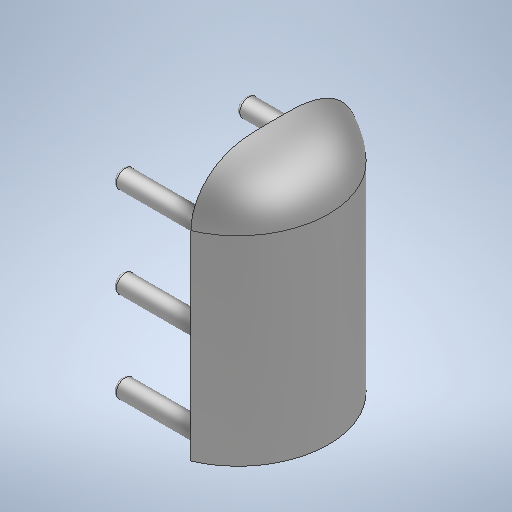
# Autodesk Inventor part: Pot Side
Saved by Autodesk Inventor 2025.2 (Build 292293000, 293)
## iProperties
Created: 2025-02-16
Part Number: Pot Side
Material: Generic
Document SubType Name: Modeling
Designer: eason
Density: 1 g/cm^3
Appearance: Anodized - Light Gray
Author: eason
Autodesk Inventor part; units mm, degrees
ref_plane "XZ Plane" through (0, 0, 0) normal (0, 1, 0) x (-1, 0, 0)
sketch "Sketch1" plane through (0, 0, 0) normal (0, 0, 1) x (1, 0, 0)
  line L0 (0, 0) -> (0, 70)
  line L1 (0, 0) -> (25, 0)
  line L2 (25, 0) -> (25, 55)
  line L3 (0, -14.6213) -> (0, 87.7279) projected
  line L4 (0, 70) -> (10, 70)
  arc A0 (25, 55) -> (10, 70) centre (10, 55) ccw
  dimension "d0" = 70
  dimension "d1" = 25
  dimension "d2" = 10
  constraints: 8 end point, 2 point on circle, 2 tangent, 2 vertical, 1 centre point, 1 horizontal, 1 perpendicular
  measures "d0" distance of L0.start L0.end
  measures "d1" distance of L0.start L1.end
  measures "d2" distance of L0.end L4.end
revolve "Revolution1" add sketch "Sketch1" angle 360 about axis through (0, -10, 0) along (0, 1, 0)
sketch "Sketch2" plane through (0, 0, 0) normal (0, -1, 0) x (1, 0, 0)
  circle A0 centre (0, 0) radius 10
  dimension "d4" = 20
  constraints: 1 centre point, 1 coincident
  measures "d4" diameter of A0
extrude "Extrusion1" cut sketch "Sketch2" against normal blind 25
sketch "Sketch3" plane through (0, 70, 0) normal (0, 1, 0) x (1, 0, 0)
  circle A0 centre (0, 0) radius 10 projected
  line L0 (10, 0) -> (-10, 0) construction
  line L1 (-35, 0) -> (35, 0) construction
  constraints: 2 end point, 2 point on circle, 1 collinear
ref_plane "Work Plane1" through (10, 70, 0) normal (1, 0, 0) x (0, 1, 0)
ref_plane "Work Plane2" through (-10, 70, 0) normal (1, 0, 0) x (0, 1, 0)
ref_plane "Work Plane3" through (0, 27.5, 25) normal (0, 0, 1) x (1, 0, 0)
sketch "Sketch4" plane through (0, 27.5, 25) normal (0, 0, 1) x (1, 0, 0)
  line L0 (10, 56.5) -> (10, -41.5) projected
  line L1 (10, 42.5) -> (-10, 42.5) projected
  arc A0 (-10, 42.5) -> (-25, 27.5) centre (-10, 27.5) ccw projected
  line L2 (-25, -27.5) -> (-25, 27.5) projected
  line L3 (25, -27.5) -> (-25, -27.5) projected
  point P0 (0, -27.5)
  point P1 (10, -27.5)
extrude "Extrusion2" cut sketch "Sketch4" against normal through all
sketch "Sketch5" plane through (10, 70, 0) normal (1, 0, 0) x (0, 1, 0)
  arc A0 (-26.2642, -10) -> (-26.2642, 10) centre (-20, 0) ccw
  line L0 (-26.2642, -10) -> (-45, -10)
  line L1 (-26.2642, 10) -> (-45, 10)
  line L2 (-84.0012, 0) -> (14.0074, 0) projected
  line L3 (-70, 22.9129) -> (-70, -22.9129) projected
  line L4 (-40.2, 0) -> (-8.2, 0) construction
  line L5 (-45, -10) -> (-45, 10)
  point P0 (-70, 0)
  dimension "d10" = 23.6
  dimension "d11" = 20
  dimension "d13" = 10
  dimension "d14" = 50
  dimension "d20" = 25
  constraints: 8 end point, 3 point on circle, 2 collinear, 2 horizontal, 1 centre point, 1 parallel, 1 point on line
  measures "d10" diameter of A0
  measures "d11" distance between parallel lines of L1 L0
  measures "d13" distance between parallel lines of L2 L0
  measures "d14" distance from line of A0.centre L3
  measures "d20" distance from line of L3 L1.end
extrude "Extrusion3" cut sketch "Sketch5" along normal blind 10
sketch "Sketch7" plane through (20, 70, 0) normal (-1, 0, 0) x (0, 0, 1)
  arc A0 (10, -26.2642) -> (-10, -26.2642) centre (0, -20) ccw projected
  circle A1 centre (0, -20) radius 11.8
  line L0 (-10, -45) -> (-10, -26.2642) projected
  line L1 (10, -26.2642) -> (10, -45) projected
  arc A2 (-10, -29.51) -> (10, -29.51) centre (0, -20) ccw
  point P0 (0, -70)
  point P1 (-10, -26.2642)
  dimension "d22" = 2
  constraints: 2 centre point, 2 concentric, 2 point on circle, 2 point on line, 1 coincident
  measures "d22" radial gap between concentric circles of A2 A1
extrude "Extrusion4" add sketch "Sketch7" along normal blind 3 contours L1 A2 L0 A1
fillet "Fillet1" radius 2 4 edges at (15, 25, -10) (15, 25, 10) (10, 25, -5) (10, 25, 5)
fillet "Fillet2" radius 1 2 edges at (17, 38.2, 0) (17, 36.2, 0)
sketch "Sketch8" plane through (0, 0, 0) normal (0, -1, 0) x (1, 0, 0)
  line L0 (10, 22.9129) -> (10, -22.9129) projected
  line L1 (10, 17) -> (15, 17)
  line L2 (15, 17) -> (15, -17)
  line L3 (15, -17) -> (10, -17)
  line L4 (10, -17) -> (10, 17)
  line L5 (-17, 0) -> (32, 0) projected
  line L6 (10, 10) -> (15, 10)
  line L7 (15, 10) -> (15, -10)
  line L8 (15, -10) -> (10, -10)
  line L9 (10, -10) -> (10, 10)
  point P0 (0, 0)
  point P1 (15, 0)
  point P2 (15, 0)
  dimension "d27" = 5
  dimension "d28" = 17
  dimension "d29" = 20
  constraints: 16 end point, 4 parallel, 4 point on line, 2 horizontal, 2 midpoint, 2 perpendicular, 1 collinear
  measures "d27" distance between parallel lines of L0 L2
  measures "d28" distance between parallel lines of L5 L1
  measures "d29" distance between parallel lines of L8 L6
sketch "Sketch9" plane through (10, 0, -22.9129) normal (-1, 0, 0) x (0, 0, 1)
  line L0 (39.9129, 0) -> (39.9129, 2.5) construction
  circle A0 centre (39.9129, 2.5) radius 2.5
  line L1 (45.8258, 0) -> (0, 0) projected
  line L2 (22.9129, -14.0012) -> (22.9129, 84.0074) projected
  circle A1 centre (5.9129, 2.5) radius 2.5
  circle A2 centre (39.9129, 27.5) radius 2.5
  circle A3 centre (5.9129, 27.5) radius 2.5
  circle A4 centre (39.9129, 52.5) radius 2.5
  circle A5 centre (5.9129, 52.5) radius 2.5
  point P0 (22.9129, 0)
  point P1 (5.9129, 0)
  dimension "d31" = 5
  dimension "d47" = 34
  dimension "d50" = 25
  constraints: 6 centre point, 2 end point, 2 vertical, 1 coincident, 1 horizontal, 1 tangent, 10 other
  measures "d31" diameter of A0
  measures "d47" distance of A0.centre A1.centre
  measures "d50" distance of A0.centre A2.centre
extrude "Extrusion5" add sketch "Sketch9" along normal blind 25
fillet "Fillet3" radius 1 6 edges at (-15, 2.5, 14.5) (-15, 2.5, -19.5) (-15, 27.5, -19.5) (-15, 27.5, 14.5) (-15, 52.5, 14.5) (-15, 52.5, -19.5)
sketch "Sketch10" plane through (0, 0, 0) normal (0, -1, 0) x (1, 0, 0)
  circle A0 centre (0, 0) radius 13
  dimension "d42" = 26
  constraints: 1 centre point, 1 coincident
  measures "d42" diameter of A0
extrude "Extrusion6" cut sketch "Sketch10" against normal blind 25
body "Solid1"
